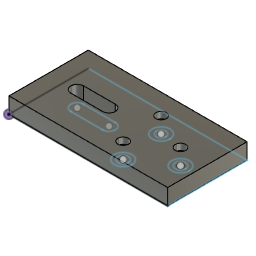
Component 1 (Autodesk Fusion 360 design; units mm, degrees)
Autodesk Fusion 360 part; units mm, degrees
note: some values were not read from the file. Set by a fixed rule: the direction of a hole.
sketch "Sketch1" plane through (0, 0, 0) normal (0, 0, 1) x (1, 0, 0)
  line L0 (0, 0) -> (100, 0)
  line L1 (100, 0) -> (100, 50)
  line L2 (100, 50) -> (0, 50)
  line L3 (0, 50) -> (0, 0)
  circle A0 centre (82.132, 25.9392) radius 5.5
  circle A1 centre (60.7017, 11.2509) radius 5.5
  circle A2 centre (58.6964, 37.1542) radius 3
  line L4 (18, 29) -> (38, 29)
  line L5 (18, 21) -> (38, 21)
  arc A3 (18, 29) -> (18, 21) centre (18, 25) ccw
  arc A4 (38, 21) -> (38, 29) centre (38, 25) ccw
  circle A5 centre (58.6964, 37.1542) radius 5.5
  circle A6 centre (60.7017, 11.2509) radius 3.3
  circle A7 centre (82.132, 25.9392) radius 3.3
  dimension "d24" = 11
  dimension "d25" = 11
  dimension "d26" = 6.6
  dimension "d27" = 11
  dimension "d28" = 6.6
  constraint horizontal L0
  constraint vertical L1
  constraint horizontal L2
  constraint vertical L3
  constraint coincident L0.start L3.end
  constraint tangent L4 A3
  constraint tangent L4 A4
  constraint tangent L5 A3
  constraint concentric A2 A5
  constraint concentric A1 A6
  constraint concentric A0 A7
  measures "d24" diameter of A5
  measures "d25" diameter of A1
  measures "d26" diameter of A6
  measures "d27" diameter of A0
  measures "d28" diameter of A7
sketch "Sketch2" plane through (0, 0, 0) normal (0, 0, 1) x (1, 0, 0)
extrude "Extrude1" add sketch "Sketch1" along normal blind 10 contours L0 L1 L2 L3 | A0 | A1 | A2 | A5 | A6 | A7
hole "Hole1" at (58.6964, 37.1542, 0) at (60.7017, 11.2509, 0) at (82.132, 25.9392, 0) direction (0, 0, 1) diameter 6.6 depth 20 tip angle 118 counterbore diameter 11 counterbore depth 6
